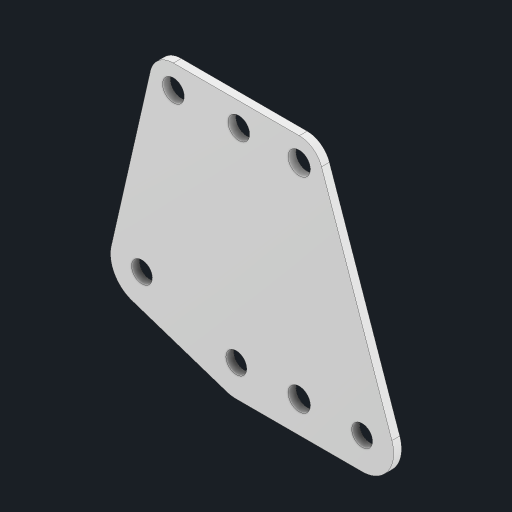
# Autodesk Inventor part: gusset
Saved by Autodesk Inventor 2024 (Build 280153000, 153)
## iProperties
Created: 2024-03-09
Part Number: gusset
Material: Acetal Resin, White
Document SubType Name: Modeling
Designer: Averey Ku
Density: 1.425 g/cm^3
Appearance: Smooth - White
Author: Averey Ku
Autodesk Inventor part; units mm, degrees
ref_plane "YZ Plane" through (0, 0, 0) normal (1, 0, 0) x (0, 1, 0)
ref_plane "XZ Plane" through (0, 0, 0) normal (0, 1, 0) x (-1, 0, 0)
ref_plane "XY Plane" through (0, 0, 0) normal (0, 0, 1) x (1, 0, 0)
sketch "main" plane through (0, 0, 0) normal (0, 0, 1) x (1, 0, 0)
  circle A0 centre (-38.8868, 18.5788) radius 2.2479
  circle A1 centre (2.3882, 18.5788) radius 2.2479
  circle A2 centre (2.3882, 43.9788) radius 2.1844
  arc A3 (3.9757, 48.4689) -> (3.4489, 48.6217) centre (2.3882, 43.9788) ccw
  arc A4 (3.9552, 14.0814) -> (7.1507, 18.5788) centre (2.3882, 18.5788) ccw
  circle A5 centre (-38.8868, 31.2788) radius 2.0955
  circle A6 centre (-38.8868, 5.8788) radius 2.0955
  arc A7 (-44.9109, 33.2868) -> (-45.2368, 31.2788) centre (-38.8868, 31.2788) ccw
  arc A8 (-45.2368, 5.8788) -> (-36.7975, -0.1177) centre (-38.8868, 5.8788) ccw
  circle A9 centre (-32.5368, 50.3288) radius 2.0955
  arc A10 (-31.1226, 56.5193) -> (-38.5609, 52.3368) centre (-32.5368, 50.3288) ccw
  line L0 (-44.9109, 33.2868) -> (-38.5609, 52.3368)
  line L1 (3.4489, 48.6217) -> (-31.1226, 56.5193)
  line L2 (3.9552, 14.0814) -> (-36.7975, -0.1177)
  line L3 (-45.2368, 31.2788) -> (-45.2368, 5.8788)
  arc A11 (7.1507, 43.9788) -> (3.4489, 48.6217) centre (2.3882, 43.9788) ccw
  line L4 (7.1507, 43.9788) -> (7.1507, 18.5788)
  circle A12 centre (2.3882, 30.7746) radius 2.1844
  point P0 (-4.3882, 4.0845)
  dimension "d11" = 4.4958
  dimension "d12" = 4.4958
  dimension "d13" = 9.525
  dimension "d14" = 9.525
  dimension "d15" = 4.191
  dimension "d16" = 4.191
  dimension "d17" = 41.275
  dimension "d18" = 41.275
  dimension "d19" = 25.4
  dimension "d20" = 4.3688
  measures "d11" diameter of A0
  measures "d12" diameter of A1
  measures "d13" diameter of A3
  measures "d14" diameter of A4
  measures "d15" diameter of A9
  measures "d16" diameter of A6
  measures "d17" horizontal distance of A5.centre A3.centre
  measures "d18" distance of A1.centre point (-38.887, 18.579)
  measures "d19" distance of A2.centre A1.centre
  measures "d20" diameter of A12
sketch "Sketch1" plane through (0, 0, 0) normal (0, 0, 1) x (1, 0, 0)
  circle A0 centre (-12.7, 0) radius 2.2479
  circle A1 centre (-12.7, 41.275) radius 2.2479
  circle A2 centre (-38.1, 41.275) radius 2.1844
  arc A3 (-42.5901, 42.8625) -> (-42.7429, 42.3356) centre (-38.1, 41.275) ccw
  arc A4 (-8.2027, 42.842) -> (-12.7, 46.0375) centre (-12.7, 41.275) ccw
  circle A5 centre (-25.4, 0) radius 2.0955
  circle A6 centre (0, 0) radius 2.0955
  arc A7 (-27.408, -6.0241) -> (-25.4, -6.35) centre (-25.4, 0) ccw
  arc A8 (0, -6.35) -> (5.9964, 2.0893) centre (0, 0) ccw
  circle A9 centre (-44.45, 6.35) radius 2.0955
  arc A10 (-50.6405, 7.7642) -> (-46.458, 0.3259) centre (-44.45, 6.35) ccw
  line L0 (-27.408, -6.0241) -> (-46.458, 0.3259)
  line L1 (-42.7429, 42.3356) -> (-50.6405, 7.7642)
  line L2 (-8.2027, 42.842) -> (5.9964, 2.0893)
  line L3 (-25.4, -6.35) -> (0, -6.35)
  arc A11 (-38.1, 46.0375) -> (-42.7429, 42.3356) centre (-38.1, 41.275) ccw
  line L4 (-38.1, 46.0375) -> (-12.7, 46.0375)
  circle A12 centre (-24.8958, 41.275) radius 2.1844
  point P0 (0, 0)
  point P1 (-42.5901, 42.8625)
  constraints: 1 other
extrude "Extrusion1" add sketch "Sketch1" along normal blind 1.5875
body "Solid1"
